Autodesk Fusion 360 part; units mm, degrees
note: some values were not read from the file. Set by a fixed rule: which sketch regions a step uses.
(part 9 of 59)
  spline S46 degree 5 poles (-3.7249, 43.2754) (-3.7256, 43.2728) (-3.7268, 43.2675) (-3.7287, 43.2596) (-3.7312, 43.2491) (-3.7343, 43.236) (-3.7374, 43.223) (-3.7405, 43.2099) (-3.7435, 43.1969) (-3.7466, 43.1839) (-3.7496, 43.171) (-3.7525, 43.158) (-3.7555, 43.1451) (-3.7584, 43.1323) (-3.7613, 43.1194) (-3.7642, 43.1066) (-3.767, 43.0938) (-3.7699, 43.081) (-3.7727, 43.0683) (-3.7755, 43.0556) (-3.7782, 43.0429) (-3.781, 43.0302) (-3.7837, 43.0176) (-3.7864, 43.005) (-3.7891, 42.9924) (-3.7917, 42.9799) (-3.7943, 42.9674) (-3.797, 42.9549) (-3.7995, 42.9424) (-3.8021, 42.93) (-3.8046, 42.9176) (-3.8071, 42.9053) (-3.8096, 42.8929) (-3.8121, 42.8806) (-3.8145, 42.8683) (-3.817, 42.8561) (-3.8194, 42.8439) (-3.8217, 42.8317) (-3.8241, 42.8195) (-3.8264, 42.8074) (-3.8288, 42.7953) (-3.831, 42.7832) (-3.8333, 42.7712) (-3.8356, 42.7592) (-3.8378, 42.7472) (-3.84, 42.7353) (-3.8422, 42.7233) (-3.8443, 42.7115) (-3.8464, 42.6996) (-3.8486, 42.6878) (-3.8507, 42.676) (-3.8527, 42.6643) (-3.8548, 42.6525) (-3.8568, 42.6409) (-3.8588, 42.6292) (-3.8608, 42.6176) (-3.8628, 42.606) (-3.8647, 42.5944) (-3.8666, 42.5829) (-3.8685, 42.5714) (-3.8704, 42.56) (-3.8722, 42.5486) (-3.8741, 42.5372) (-3.8759, 42.5258) (-3.8777, 42.5145) (-3.8795, 42.5032) (-3.8812, 42.492) (-3.8829, 42.4807) (-3.8846, 42.4696) (-3.8863, 42.4584) (-3.888, 42.4473) (-3.8896, 42.4362) (-3.8913, 42.4252) (-3.8929, 42.4142) (-3.8945, 42.4032) (-3.896, 42.3923) (-3.8976, 42.3814) (-3.8991, 42.3705) (-3.9006, 42.3597) (-3.9021, 42.3489) (-3.9035, 42.3382) (-3.905, 42.3274) (-3.9064, 42.3168) (-3.9078, 42.3061) (-3.9092, 42.2955) (-3.9106, 42.285) (-3.9119, 42.2744) (-3.9132, 42.264) (-3.9145, 42.2535) (-3.9158, 42.2431) (-3.9171, 42.2327) (-3.9183, 42.2224) (-3.9196, 42.2121) (-3.9208, 42.2018) (-3.922, 42.1916) (-3.9231, 42.1814) (-3.9243, 42.1713) (-3.9254, 42.1612) (-3.9265, 42.1512) (-3.9276, 42.1411) (-3.9287, 42.1312) (-3.9297, 42.1212) (-3.9308, 42.1113) (-3.9318, 42.1015) (-3.9328, 42.0917) (-3.9338, 42.0819) (-3.9348, 42.0722) (-3.9357, 42.0625) (-3.9366, 42.0529) (-3.9375, 42.0433) (-3.9384, 42.0337) (-3.9393, 42.0242) (-3.9402, 42.0147) (-3.941, 42.0053) (-3.9418, 41.9959) (-3.9426, 41.9866) (-3.9434, 41.9773) (-3.9442, 41.968) (-3.9449, 41.9588) (-3.9457, 41.9497) (-3.9464, 41.9406) (-3.9471, 41.9315) (-3.9478, 41.9225) (-3.9484, 41.9135) (-3.9491, 41.9045) (-3.9497, 41.8957) (-3.9503, 41.8868) (-3.9509, 41.878) (-3.9515, 41.8693) (-3.9521, 41.8606) (-3.9526, 41.8519) (-3.9532, 41.8433) (-3.9537, 41.8348) (-3.9542, 41.8263) (-3.9547, 41.8178) (-3.9552, 41.8094) (-3.9556, 41.801) (-3.9561, 41.7927) (-3.9565, 41.7845) (-3.9569, 41.7763) (-3.9573, 41.7681) (-3.9577, 41.76) (-3.9581, 41.7519) (-3.9584, 41.7439) (-3.9588, 41.736) (-3.9591, 41.7281) (-3.9594, 41.7202) (-3.9597, 41.7124) (-3.96, 41.7047) (-3.9603, 41.697) (-3.9605, 41.6893) (-3.9607, 41.6817) (-3.961, 41.6742) (-3.9612, 41.6667) (-3.9614, 41.6593) (-3.9616, 41.6519) (-3.9618, 41.6446) (-3.9619, 41.6374) (-3.9621, 41.6302) (-3.9622, 41.623) (-3.9623, 41.6159) (-3.9625, 41.6089) (-3.9626, 41.6019) (-3.9626, 41.595) (-3.9627, 41.5882) (-3.9628, 41.5814) (-3.9628, 41.5746) (-3.9629, 41.568) (-3.9629, 41.5613) (-3.9629, 41.5548) (-3.963, 41.5483) (-3.963, 41.5418) (-3.9629, 41.5355) (-3.9629, 41.5291) (-3.9629, 41.5229) (-3.9629, 41.5167) (-3.9628, 41.5106) (-3.9627, 41.5045) (-3.9627, 41.4985) (-3.9626, 41.4926) (-3.9625, 41.4867) (-3.9624, 41.4809) (-3.9623, 41.4752) (-3.9622, 41.4695) (-3.9621, 41.4639) (-3.962, 41.4584) (-3.9618, 41.4529) (-3.9617, 41.4475) (-3.9615, 41.4422) (-3.9614, 41.4369) (-3.9612, 41.4317) (-3.961, 41.4266) (-3.9609, 41.4215) (-3.9607, 41.4166) (-3.9605, 41.4117) (-3.9603, 41.4068) (-3.9601, 41.4021) (-3.9599, 41.3974) (-3.9597, 41.3928) (-3.9595, 41.3882) (-3.9593, 41.3838) (-3.959, 41.3794) (-3.9588, 41.3751) (-3.9586, 41.3709) (-3.9584, 41.3667) (-3.9581, 41.3626) (-3.9579, 41.3586) (-3.9577, 41.3547) (-3.9574, 41.3509) (-3.9572, 41.3472) (-3.9569, 41.3435) (-3.9567, 41.3399) (-3.9564, 41.3364) (-3.9562, 41.333) (-3.9559, 41.3297) (-3.9557, 41.3264) (-3.9555, 41.3233) (-3.9552, 41.3202) (-3.955, 41.3172) (-3.9547, 41.3144) (-3.9545, 41.3116) (-3.9543, 41.3089) (-3.954, 41.3063) (-3.9538, 41.3037) (-3.9536, 41.3013) (-3.9534, 41.299) (-3.9531, 41.2968) (-3.9529, 41.2946) (-3.9527, 41.2926) (-3.9525, 41.2907) (-3.9523, 41.2889) (-3.9522, 41.2871) (-3.952, 41.2855) (-3.9518, 41.284) (-3.9517, 41.2826) (-3.9515, 41.2813) (-3.9514, 41.2801) (-3.9512, 41.279) (-3.9511, 41.278) (-3.951, 41.2772) (-3.9509, 41.2764) (-3.9509, 41.2759) (-3.9508, 41.2756) (-3.9508, 41.2754) (-3.9508, 41.2753) knots -1 -1 -1 -1 -1 -1 -0.99583333 -0.99166667 -0.9875 -0.98333333 -0.97916667 -0.975 -0.97083333 -0.96666667 -0.9625 -0.95833333 -0.95416667 -0.95 -0.94583333 -0.94166667 -0.9375 -0.93333333 -0.92916667 -0.925 -0.92083333 -0.91666667 -0.9125 -0.90833333 -0.90416667 -0.9 -0.89583333 -0.89166667 -0.8875 -0.88333333 -0.87916667 -0.875 -0.87083333 -0.86666667 -0.8625 -0.85833333 -0.85416667 -0.85 -0.84583333 -0.84166667 -0.8375 -0.83333333 -0.82916667 -0.825 -0.82083333 -0.81666667 -0.8125 -0.80833333 -0.80416667 -0.8 -0.79583333 -0.79166667 -0.7875 -0.78333333 -0.77916667 -0.775 -0.77083333 -0.76666667 -0.7625 -0.75833333 -0.75416667 -0.75 -0.74583333 -0.74166667 -0.7375 -0.73333333 -0.72916667 -0.725 -0.72083333 -0.71666667 -0.7125 -0.70833333 -0.70416667 -0.7 -0.69583333 -0.69166667 -0.6875 -0.68333333 -0.67916667 -0.675 -0.67083333 -0.66666667 -0.6625 -0.65833333 -0.65416667 -0.65 -0.64583333 -0.64166667 -0.6375 -0.63333333 -0.62916667 -0.625 -0.62083333 -0.61666667 -0.6125 -0.60833333 -0.60416667 -0.6 -0.59583333 -0.59166667 -0.5875 -0.58333333 -0.57916667 -0.575 -0.57083333 -0.56666667 -0.5625 -0.55833333 -0.55416667 -0.55 -0.54583333 -0.54166667 -0.5375 -0.53333333 -0.52916667 -0.525 -0.52083333 -0.51666667 -0.5125 -0.50833333 -0.50416667 -0.5 -0.49583333 -0.49166667 -0.4875 -0.48333333 -0.47916667 -0.475 -0.47083333 -0.46666667 -0.4625 -0.45833333 -0.45416667 -0.45 -0.44583333 -0.44166667 -0.4375 -0.43333333 -0.42916667 -0.425 -0.42083333 -0.41666667 -0.4125 -0.40833333 -0.40416667 -0.4 -0.39583333 -0.39166667 -0.3875 -0.38333333 -0.37916667 -0.375 -0.37083333 -0.36666667 -0.3625 -0.35833333 -0.35416667 -0.35 -0.34583333 -0.34166667 -0.3375 -0.33333333 -0.32916667 -0.325 -0.32083333 -0.31666667 -0.3125 -0.30833333 -0.30416667 -0.3 -0.29583333 -0.29166667 -0.2875 -0.28333333 -0.27916667 -0.275 -0.27083333 -0.26666667 -0.2625 -0.25833333 -0.25416667 -0.25 -0.24583333 -0.24166667 -0.2375 -0.23333333 -0.22916667 -0.225 -0.22083333 -0.21666667 -0.2125 -0.20833333 -0.20416667 -0.2 -0.19583333 -0.19166667 -0.1875 -0.18333333 -0.17916667 -0.175 -0.17083333 -0.16666667 -0.1625 -0.15833333 -0.15416667 -0.15 -0.14583333 -0.14166667 -0.1375 -0.13333333 -0.12916667 -0.125 -0.12083333 -0.11666667 -0.1125 -0.10833333 -0.10416667 -0.1 -0.09583333 -0.09166667 -0.0875 -0.08333333 -0.07916667 -0.075 -0.07083333 -0.06666667 -0.0625 -0.05833333 -0.05416667 -0.05 -0.04583333 -0.04166667 -0.0375 -0.03333333 -0.02916667 -0.025 -0.02083333 -0.01666667 -0.0125 -0.00833333 -0.00416667 0 0 0 0 0 0
  spline S47 degree 5 poles (-21.1029, 35.2084) (-21.1018, 35.2059) (-21.0998, 35.2009) (-21.0967, 35.1934) (-21.0925, 35.1834) (-21.0873, 35.171) (-21.0822, 35.1586) (-21.077, 35.1462) (-21.0718, 35.1339) (-21.0666, 35.1217) (-21.0614, 35.1094) (-21.0562, 35.0972) (-21.051, 35.085) (-21.0458, 35.0729) (-21.0406, 35.0608) (-21.0354, 35.0487) (-21.0302, 35.0367) (-21.025, 35.0247) (-21.0198, 35.0127) (-21.0145, 35.0008) (-21.0093, 34.9889) (-21.0041, 34.9771) (-20.9989, 34.9653) (-20.9937, 34.9535) (-20.9884, 34.9417) (-20.9832, 34.93) (-20.978, 34.9184) (-20.9727, 34.9067) (-20.9675, 34.8951) (-20.9623, 34.8836) (-20.957, 34.8721) (-20.9518, 34.8606) (-20.9466, 34.8491) (-20.9413, 34.8377) (-20.9361, 34.8264) (-20.9308, 34.815) (-20.9256, 34.8037) (-20.9204, 34.7925) (-20.9151, 34.7812) (-20.9099, 34.7701) (-20.9046, 34.7589) (-20.8994, 34.7478) (-20.8942, 34.7367) (-20.8889, 34.7257) (-20.8837, 34.7147) (-20.8784, 34.7038) (-20.8732, 34.6928) (-20.868, 34.682) (-20.8627, 34.6711) (-20.8575, 34.6603) (-20.8523, 34.6496) (-20.847, 34.6388) (-20.8418, 34.6281) (-20.8366, 34.6175) (-20.8313, 34.6069) (-20.8261, 34.5963) (-20.8209, 34.5858) (-20.8157, 34.5753) (-20.8105, 34.5649) (-20.8052, 34.5544) (-20.8, 34.5441) (-20.7948, 34.5337) (-20.7896, 34.5235) (-20.7844, 34.5132) (-20.7792, 34.503) (-20.774, 34.4928) (-20.7688, 34.4827) (-20.7636, 34.4726) (-20.7584, 34.4625) (-20.7532, 34.4525) (-20.748, 34.4426) (-20.7429, 34.4326) (-20.7377, 34.4228) (-20.7325, 34.4129) (-20.7274, 34.4031) (-20.7222, 34.3933) (-20.717, 34.3836) (-20.7119, 34.3739) (-20.7067, 34.3643) (-20.7016, 34.3547) (-20.6965, 34.3451) (-20.6913, 34.3356) (-20.6862, 34.3261) (-20.6811, 34.3167) (-20.676, 34.3073) (-20.6709, 34.298) (-20.6658, 34.2887) (-20.6607, 34.2794) (-20.6556, 34.2702) (-20.6505, 34.261) (-20.6454, 34.2519) (-20.6404, 34.2428) (-20.6353, 34.2337) (-20.6303, 34.2247) (-20.6252, 34.2158) (-20.6202, 34.2068) (-20.6152, 34.198) (-20.6101, 34.1891) (-20.6051, 34.1803) (-20.6001, 34.1716) (-20.5951, 34.1629) (-20.5902, 34.1542) (-20.5852, 34.1456) (-20.5802, 34.1371) (-20.5753, 34.1285) (-20.5703, 34.1201) (-20.5654, 34.1116) (-20.5605, 34.1032) (-20.5555, 34.0949) (-20.5506, 34.0866) (-20.5457, 34.0783) (-20.5409, 34.0701) (-20.536, 34.0619) (-20.5311, 34.0538) (-20.5263, 34.0458) (-20.5214, 34.0377) (-20.5166, 34.0297) (-20.5118, 34.0218) (-20.507, 34.0139) (-20.5022, 34.0061) (-20.4974, 33.9983) (-20.4927, 33.9905) (-20.4879, 33.9828) (-20.4832, 33.9752) (-20.4784, 33.9676) (-20.4737, 33.96) (-20.469, 33.9525) (-20.4644, 33.945) (-20.4597, 33.9376) (-20.455, 33.9302) (-20.4504, 33.9229) (-20.4458, 33.9156) (-20.4412, 33.9084) (-20.4366, 33.9012) (-20.432, 33.8941) (-20.4274, 33.887) (-20.4229, 33.88) (-20.4184, 33.873) (-20.4139, 33.8661) (-20.4094, 33.8592) (-20.4049, 33.8523) (-20.4004, 33.8455) (-20.396, 33.8388) (-20.3916, 33.8321) (-20.3872, 33.8255) (-20.3828, 33.8189) (-20.3784, 33.8124) (-20.3741, 33.8059) (-20.3698, 33.7995) (-20.3655, 33.7931) (-20.3612, 33.7867) (-20.3569, 33.7805) (-20.3527, 33.7742) (-20.3484, 33.7681) (-20.3442, 33.7619) (-20.3401, 33.7559) (-20.3359, 33.7498) (-20.3318, 33.7439) (-20.3277, 33.738) (-20.3236, 33.7321) (-20.3195, 33.7263) (-20.3155, 33.7205) (-20.3115, 33.7148) (-20.3075, 33.7092) (-20.3035, 33.7036) (-20.2996, 33.6981) (-20.2956, 33.6926) (-20.2918, 33.6871) (-20.2879, 33.6818) (-20.2841, 33.6764) (-20.2802, 33.6712) (-20.2765, 33.666) (-20.2727, 33.6608) (-20.269, 33.6557) (-20.2653, 33.6507) (-20.2616, 33.6457) (-20.258, 33.6408) (-20.2544, 33.6359) (-20.2508, 33.6311) (-20.2472, 33.6263) (-20.2437, 33.6216) (-20.2402, 33.617) (-20.2368, 33.6124) (-20.2333, 33.6079) (-20.23, 33.6034) (-20.2266, 33.599) (-20.2233, 33.5947) (-20.22, 33.5904) (-20.2167, 33.5862) (-20.2135, 33.582) (-20.2103, 33.5779) (-20.2072, 33.5739) (-20.2041, 33.5699) (-20.201, 33.566) (-20.198, 33.5621) (-20.195, 33.5583) (-20.192, 33.5546) (-20.1891, 33.5509) (-20.1862, 33.5473) (-20.1834, 33.5437) (-20.1806, 33.5403) (-20.1778, 33.5368) (-20.1751, 33.5335) (-20.1724, 33.5302) (-20.1698, 33.527) (-20.1672, 33.5238) (-20.1647, 33.5207) (-20.1622, 33.5177) (-20.1597, 33.5148) (-20.1573, 33.5119) (-20.155, 33.509) (-20.1527, 33.5063) (-20.1504, 33.5036) (-20.1482, 33.501) (-20.1461, 33.4984) (-20.144, 33.496) (-20.1419, 33.4936) (-20.1399, 33.4912) (-20.138, 33.489) (-20.1361, 33.4868) (-20.1343, 33.4847) (-20.1325, 33.4826) (-20.1308, 33.4806) (-20.1291, 33.4787) (-20.1275, 33.4769) (-20.126, 33.4752) (-20.1245, 33.4735) (-20.123, 33.4719) (-20.1217, 33.4704) (-20.1204, 33.4689) (-20.1192, 33.4675) (-20.118, 33.4663) (-20.1169, 33.4651) (-20.1159, 33.4639) (-20.1149, 33.4629) (-20.114, 33.4619) (-20.1132, 33.461) (-20.1125, 33.4602) (-20.1118, 33.4595) (-20.1112, 33.4589) (-20.1107, 33.4583) (-20.1104, 33.458) (-20.1102, 33.4577) (-20.11, 33.4576) (-20.11, 33.4575) knots -1 -1 -1 -1 -1 -1 -0.99583333 -0.99166667 -0.9875 -0.98333333 -0.97916667 -0.975 -0.97083333 -0.96666667 -0.9625 -0.95833333 -0.95416667 -0.95 -0.94583333 -0.94166667 -0.9375 -0.93333333 -0.92916667 -0.925 -0.92083333 -0.91666667 -0.9125 -0.90833333 -0.90416667 -0.9 -0.89583333 -0.89166667 -0.8875 -0.88333333 -0.87916667 -0.875 -0.87083333 -0.86666667 -0.8625 -0.85833333 -0.85416667 -0.85 -0.84583333 -0.84166667 -0.8375 -0.83333333 -0.82916667 -0.825 -0.82083333 -0.81666667 -0.8125 -0.80833333 -0.80416667 -0.8 -0.79583333 -0.79166667 -0.7875 -0.78333333 -0.77916667 -0.775 -0.77083333 -0.76666667 -0.7625 -0.75833333 -0.75416667 -0.75 -0.74583333 -0.74166667 -0.7375 -0.73333333 -0.72916667 -0.725 -0.72083333 -0.71666667 -0.7125 -0.70833333 -0.70416667 -0.7 -0.69583333 -0.69166667 -0.6875 -0.68333333 -0.67916667 -0.675 -0.67083333 -0.66666667 -0.6625 -0.65833333 -0.65416667 -0.65 -0.64583333 -0.64166667 -0.6375 -0.63333333 -0.62916667 -0.625 -0.62083333 -0.61666667 -0.6125 -0.60833333 -0.60416667 -0.6 -0.59583333 -0.59166667 -0.5875 -0.58333333 -0.57916667 -0.575 -0.57083333 -0.56666667 -0.5625 -0.55833333 -0.55416667 -0.55 -0.54583333 -0.54166667 -0.5375 -0.53333333 -0.52916667 -0.525 -0.52083333 -0.51666667 -0.5125 -0.50833333 -0.50416667 -0.5 -0.49583333 -0.49166667 -0.4875 -0.48333333 -0.47916667 -0.475 -0.47083333 -0.46666667 -0.4625 -0.45833333 -0.45416667 -0.45 -0.44583333 -0.44166667 -0.4375 -0.43333333 -0.42916667 -0.425 -0.42083333 -0.41666667 -0.4125 -0.40833333 -0.40416667 -0.4 -0.39583333 -0.39166667 -0.3875 -0.38333333 -0.37916667 -0.375 -0.37083333 -0.36666667 -0.3625 -0.35833333 -0.35416667 -0.35 -0.34583333 -0.34166667 -0.3375 -0.33333333 -0.32916667 -0.325 -0.32083333 -0.31666667 -0.3125 -0.30833333 -0.30416667 -0.3 -0.29583333 -0.29166667 -0.2875 -0.28333333 -0.27916667 -0.275 -0.27083333 -0.26666667 -0.2625 -0.25833333 -0.25416667 -0.25 -0.24583333 -0.24166667 -0.2375 -0.23333333 -0.22916667 -0.225 -0.22083333 -0.21666667 -0.2125 -0.20833333 -0.20416667 -0.2 -0.19583333 -0.19166667 -0.1875 -0.18333333 -0.17916667 -0.175 -0.17083333 -0.16666667 -0.1625 -0.15833333 -0.15416667 -0.15 -0.14583333 -0.14166667 -0.1375 -0.13333333 -0.12916667 -0.125 -0.12083333 -0.11666667 -0.1125 -0.10833333 -0.10416667 -0.1 -0.09583333 -0.09166667 -0.0875 -0.08333333 -0.07916667 -0.075 -0.07083333 -0.06666667 -0.0625 -0.05833333 -0.05416667 -0.05 -0.04583333 -0.04166667 -0.0375 -0.03333333 -0.02916667 -0.025 -0.02083333 -0.01666667 -0.0125 -0.00833333 -0.00416667 0 0 0 0 0 0
  spline S48 degree 5 poles (-20.11, -8.4575) (-20.11, -8.4576) (-20.1102, -8.4577) (-20.1104, -8.458) (-20.1107, -8.4583) (-20.1112, -8.4589) (-20.1118, -8.4595) (-20.1125, -8.4602) (-20.1132, -8.461) (-20.114, -8.4619) (-20.1149, -8.4629) (-20.1159, -8.4639) (-20.1169, -8.4651) (-20.118, -8.4663) (-20.1192, -8.4675) (-20.1204, -8.4689) (-20.1217, -8.4704) (-20.123, -8.4719) (-20.1245, -8.4735) (-20.126, -8.4752) (-20.1275, -8.4769) (-20.1291, -8.4787) (-20.1308, -8.4806) (-20.1325, -8.4826) (-20.1343, -8.4847) (-20.1361, -8.4868) (-20.138, -8.489) (-20.1399, -8.4912) (-20.1419, -8.4936) (-20.144, -8.496) (-20.1461, -8.4984) (-20.1482, -8.501) (-20.1504, -8.5036) (-20.1527, -8.5063) (-20.155, -8.509) (-20.1573, -8.5119) (-20.1597, -8.5148) (-20.1622, -8.5177) (-20.1647, -8.5207) (-20.1672, -8.5238) (-20.1698, -8.527) (-20.1724, -8.5302) (-20.1751, -8.5335) (-20.1778, -8.5368) (-20.1806, -8.5403) (-20.1834, -8.5437) (-20.1862, -8.5473) (-20.1891, -8.5509) (-20.192, -8.5546) (-20.195, -8.5583) (-20.198, -8.5621) (-20.201, -8.566) (-20.2041, -8.5699) (-20.2072, -8.5739) (-20.2103, -8.5779) (-20.2135, -8.582) (-20.2167, -8.5862) (-20.22, -8.5904) (-20.2233, -8.5947) (-20.2266, -8.599) (-20.23, -8.6034) (-20.2333, -8.6079) (-20.2368, -8.6124) (-20.2402, -8.617) (-20.2437, -8.6216) (-20.2472, -8.6263) (-20.2508, -8.6311) (-20.2544, -8.6359) (-20.258, -8.6408) (-20.2616, -8.6457) (-20.2653, -8.6507) (-20.269, -8.6557) (-20.2727, -8.6608) (-20.2765, -8.666) (-20.2802, -8.6712) (-20.2841, -8.6764) (-20.2879, -8.6818) (-20.2918, -8.6871) (-20.2956, -8.6926) (-20.2996, -8.6981) (-20.3035, -8.7036) (-20.3075, -8.7092) (-20.3115, -8.7148) (-20.3155, -8.7205) (-20.3195, -8.7263) (-20.3236, -8.7321) (-20.3277, -8.738) (-20.3318, -8.7439) (-20.3359, -8.7498) (-20.3401, -8.7559) (-20.3442, -8.7619) (-20.3484, -8.7681) (-20.3527, -8.7742) (-20.3569, -8.7805) (-20.3612, -8.7867) (-20.3655, -8.7931) (-20.3698, -8.7995) (-20.3741, -8.8059) (-20.3784, -8.8124) (-20.3828, -8.8189) (-20.3872, -8.8255) (-20.3916, -8.8321) (-20.396, -8.8388) (-20.4004, -8.8455) (-20.4049, -8.8523) (-20.4094, -8.8592) (-20.4139, -8.8661) (-20.4184, -8.873) (-20.4229, -8.88) (-20.4274, -8.887) (-20.432, -8.8941) (-20.4366, -8.9012) (-20.4412, -8.9084) (-20.4458, -8.9156) (-20.4504, -8.9229) (-20.455, -8.9302) (-20.4597, -8.9376) (-20.4644, -8.945) (-20.469, -8.9525) (-20.4737, -8.96) (-20.4784, -8.9676) (-20.4832, -8.9752) (-20.4879, -8.9828) (-20.4927, -8.9905) (-20.4974, -8.9983) (-20.5022, -9.0061) (-20.507, -9.0139) (-20.5118, -9.0218) (-20.5166, -9.0297) (-20.5214, -9.0377) (-20.5263, -9.0458) (-20.5311, -9.0538) (-20.536, -9.0619) (-20.5409, -9.0701) (-20.5457, -9.0783) (-20.5506, -9.0866) (-20.5555, -9.0949) (-20.5605, -9.1032) (-20.5654, -9.1116) (-20.5703, -9.1201) (-20.5753, -9.1285) (-20.5802, -9.1371) (-20.5852, -9.1456) (-20.5902, -9.1542) (-20.5951, -9.1629) (-20.6001, -9.1716) (-20.6051, -9.1803) (-20.6101, -9.1891) (-20.6152, -9.198) (-20.6202, -9.2068) (-20.6252, -9.2158) (-20.6303, -9.2247) (-20.6353, -9.2337) (-20.6404, -9.2428) (-20.6454, -9.2519) (-20.6505, -9.261) (-20.6556, -9.2702) (-20.6607, -9.2794) (-20.6658, -9.2887) (-20.6709, -9.298) (-20.676, -9.3073) (-20.6811, -9.3167) (-20.6862, -9.3261) (-20.6913, -9.3356) (-20.6965, -9.3451) (-20.7016, -9.3547) (-20.7067, -9.3643) (-20.7119, -9.3739) (-20.717, -9.3836) (-20.7222, -9.3933) (-20.7274, -9.4031) (-20.7325, -9.4129) (-20.7377, -9.4228) (-20.7429, -9.4326) (-20.748, -9.4426) (-20.7532, -9.4525) (-20.7584, -9.4625) (-20.7636, -9.4726) (-20.7688, -9.4827) (-20.774, -9.4928) (-20.7792, -9.503) (-20.7844, -9.5132) (-20.7896, -9.5235) (-20.7948, -9.5337) (-20.8, -9.5441) (-20.8052, -9.5544) (-20.8105, -9.5649) (-20.8157, -9.5753) (-20.8209, -9.5858) (-20.8261, -9.5963) (-20.8313, -9.6069) (-20.8366, -9.6175) (-20.8418, -9.6281) (-20.847, -9.6388) (-20.8523, -9.6496) (-20.8575, -9.6603) (-20.8627, -9.6711) (-20.868, -9.682) (-20.8732, -9.6928) (-20.8784, -9.7038) (-20.8837, -9.7147) (-20.8889, -9.7257) (-20.8942, -9.7367) (-20.8994, -9.7478) (-20.9046, -9.7589) (-20.9099, -9.7701) (-20.9151, -9.7812) (-20.9204, -9.7925) (-20.9256, -9.8037) (-20.9308, -9.815) (-20.9361, -9.8264) (-20.9413, -9.8377) (-20.9466, -9.8491) (-20.9518, -9.8606) (-20.957, -9.8721) (-20.9623, -9.8836) (-20.9675, -9.8951) (-20.9727, -9.9067) (-20.978, -9.9184) (-20.9832, -9.93) (-20.9884, -9.9417) (-20.9937, -9.9535) (-20.9989, -9.9653) (-21.0041, -9.9771) (-21.0093, -9.9889) (-21.0145, -10.0008) (-21.0198, -10.0127) (-21.025, -10.0247) (-21.0302, -10.0367) (-21.0354, -10.0487) (-21.0406, -10.0608) (-21.0458, -10.0729) (-21.051, -10.085) (-21.0562, -10.0972) (-21.0614, -10.1094) (-21.0666, -10.1217) (-21.0718, -10.1339) (-21.077, -10.1462) (-21.0822, -10.1586) (-21.0873, -10.171) (-21.0925, -10.1834) (-21.0967, -10.1934) (-21.0998, -10.2009) (-21.1018, -10.2059) (-21.1029, -10.2084) knots 0 0 0 0 0 0 0.00416667 0.00833333 0.0125 0.01666667 0.02083333 0.025 0.02916667 0.03333333 0.0375 0.04166667 0.04583333 0.05 0.05416667 0.05833333 0.0625 0.06666667 0.07083333 0.075 0.07916667 0.08333333 0.0875 0.09166667 0.09583333 0.1 0.10416667 0.10833333 0.1125 0.11666667 0.12083333 0.125 0.12916667 0.13333333 0.1375 0.14166667 0.14583333 0.15 0.15416667 0.15833333 0.1625 0.16666667 0.17083333 0.175 0.17916667 0.18333333 0.1875 0.19166667 0.19583333 0.2 0.20416667 0.20833333 0.2125 0.21666667 0.22083333 0.225 0.22916667 0.23333333 0.2375 0.24166667 0.24583333 0.25 0.25416667 0.25833333 0.2625 0.26666667 0.27083333 0.275 0.27916667 0.28333333 0.2875 0.29166667 0.29583333 0.3 0.30416667 0.30833333 0.3125 0.31666667 0.32083333 0.325 0.32916667 0.33333333 0.3375 0.34166667 0.34583333 0.35 0.35416667 0.35833333 0.3625 0.36666667 0.37083333 0.375 0.37916667 0.38333333 0.3875 0.39166667 0.39583333 0.4 0.40416667 0.40833333 0.4125 0.41666667 0.42083333 0.425 0.42916667 0.43333333 0.4375 0.44166667 0.44583333 0.45 0.45416667 0.45833333 0.4625 0.46666667 0.47083333 0.475 0.47916667 0.48333333 0.4875 0.49166667 0.49583333 0.5 0.50416667 0.50833333 0.5125 0.51666667 0.52083333 0.525 0.52916667 0.53333333 0.5375 0.54166667 0.54583333 0.55 0.55416667 0.55833333 0.5625 0.56666667 0.57083333 0.575 0.57916667 0.58333333 0.5875 0.59166667 0.59583333 0.6 0.60416667 0.60833333 0.6125 0.61666667 0.62083333 0.625 0.62916667 0.63333333 0.6375 0.64166667 0.64583333 0.65 0.65416667 0.65833333 0.6625 0.66666667 0.67083333 0.675 0.67916667 0.68333333 0.6875 0.69166667 0.69583333 0.7 0.70416667 0.70833333 0.7125 0.71666667 0.72083333 0.725 0.72916667 0.73333333 0.7375 0.74166667 0.74583333 0.75 0.75416667 0.75833333 0.7625 0.76666667 0.77083333 0.775 0.77916667 0.78333333 0.7875 0.79166667 0.79583333 0.8 0.80416667 0.80833333 0.8125 0.81666667 0.82083333 0.825 0.82916667 0.83333333 0.8375 0.84166667 0.84583333 0.85 0.85416667 0.85833333 0.8625 0.86666667 0.87083333 0.875 0.87916667 0.88333333 0.8875 0.89166667 0.89583333 0.9 0.90416667 0.90833333 0.9125 0.91666667 0.92083333 0.925 0.92916667 0.93333333 0.9375 0.94166667 0.94583333 0.95 0.95416667 0.95833333 0.9625 0.96666667 0.97083333 0.975 0.97916667 0.98333333 0.9875 0.99166667 0.99583333 1 1 1 1 1 1
  line L118 (-8.0125, 40.1109) -> (-8.0945, 40.3937)
  arc A63 (-5.9675, 42.9202) -> (-6.9214, 42.7174) centre (0, 12.5) ccw
  line L119 (-6.9368, 40.7039) -> (-6.8665, 40.418)
  arc A64 (-9.7471, 39.5473) -> (-10.8547, 39.1221) centre (0, 12.5) ccw
  spline S49 degree 5 poles (-10.9662, 39.3955) (-10.9662, 39.3956) (-10.9663, 39.3958) (-10.9664, 39.3961) (-10.9666, 39.3966) (-10.9669, 39.3973) (-10.9672, 39.3981) (-10.9676, 39.399) (-10.9681, 39.4) (-10.9685, 39.4011) (-10.9691, 39.4023) (-10.9696, 39.4036) (-10.9702, 39.405) (-10.9709, 39.4065) (-10.9716, 39.408) (-10.9724, 39.4097) (-10.9731, 39.4115) (-10.974, 39.4134) (-10.9749, 39.4153) (-10.9758, 39.4173) (-10.9768, 39.4195) (-10.9778, 39.4217) (-10.9788, 39.424) (-10.9799, 39.4263) (-10.9811, 39.4288) (-10.9823, 39.4313) (-10.9835, 39.4339) (-10.9848, 39.4366) (-10.9861, 39.4394) (-10.9875, 39.4423) (-10.9889, 39.4452) (-10.9903, 39.4482) (-10.9918, 39.4513) (-10.9934, 39.4544) (-10.9949, 39.4577) (-10.9966, 39.461) (-10.9982, 39.4643) (-10.9999, 39.4678) (-11.0017, 39.4713) (-11.0035, 39.4748) (-11.0053, 39.4785) (-11.0072, 39.4822) (-11.0091, 39.486) (-11.0111, 39.4898) (-11.0131, 39.4937) (-11.0151, 39.4977) (-11.0172, 39.5017) (-11.0193, 39.5058) (-11.0215, 39.51) (-11.0237, 39.5142) (-11.0259, 39.5185) (-11.0282, 39.5228) (-11.0306, 39.5272) (-11.0329, 39.5317) (-11.0353, 39.5362) (-11.0378, 39.5408) (-11.0403, 39.5454) (-11.0428, 39.5501) (-11.0454, 39.5549) (-11.048, 39.5597) (-11.0507, 39.5645) (-11.0534, 39.5694) (-11.0561, 39.5744) (-11.0589, 39.5794) (-11.0617, 39.5845) (-11.0646, 39.5896) (-11.0675, 39.5948) (-11.0704, 39.6) (-11.0734, 39.6053) (-11.0764, 39.6106) (-11.0795, 39.616) (-11.0826, 39.6214) (-11.0857, 39.6269) (-11.0889, 39.6324) (-11.0921, 39.638) (-11.0954, 39.6436) (-11.0987, 39.6493) (-11.102, 39.655) (-11.1054, 39.6608) (-11.1088, 39.6666) (-11.1123, 39.6725) (-11.1158, 39.6784) (-11.1193, 39.6843) (-11.1229, 39.6903) (-11.1265, 39.6963) (-11.1301, 39.7024) (-11.1338, 39.7085) (-11.1376, 39.7147) (-11.1413, 39.7209) (-11.1451, 39.7271) (-11.149, 39.7334) (-11.1529, 39.7397) (-11.1568, 39.7461) (-11.1608, 39.7525) (-11.1648, 39.759) (-11.1688, 39.7654) (-11.1729, 39.772) (-11.177, 39.7785) (-11.1812, 39.7851) (-11.1854, 39.7918) (-11.1896, 39.7985) (-11.1939, 39.8052) (-11.1982, 39.8119) (-11.2025, 39.8187) (-11.2069, 39.8256) (-11.2113, 39.8324) (-11.2158, 39.8393) (-11.2203, 39.8463) (-11.2248, 39.8533) (-11.2294, 39.8603) (-11.234, 39.8673) (-11.2387, 39.8744) (-11.2434, 39.8815) (-11.2481, 39.8887) (-11.2529, 39.8958) (-11.2577, 39.9031) (-11.2625, 39.9103) (-11.2674, 39.9176) (-11.2723, 39.9249) (-11.2773, 39.9323) (-11.2823, 39.9396) (-11.2873, 39.947) (-11.2924, 39.9545) (-11.2975, 39.962) (-11.3026, 39.9695) (-11.3078, 39.977) (-11.313, 39.9846) (-11.3183, 39.9922) (-11.3235, 39.9998) (-11.3289, 40.0074) (-11.3342, 40.0151) (-11.3396, 40.0228) (-11.3451, 40.0306) (-11.3506, 40.0384) (-11.3561, 40.0462) (-11.3616, 40.054) (-11.3672, 40.0618) (-11.3728, 40.0697) (-11.3785, 40.0776) (-11.3842, 40.0856) (-11.3899, 40.0936) (-11.3957, 40.1015) (-11.4015, 40.1096) (-11.4074, 40.1176) (-11.4132, 40.1257) (-11.4192, 40.1338) (-11.4251, 40.1419) (-11.4311, 40.1501) (-11.4371, 40.1582) (-11.4432, 40.1665) (-11.4493, 40.1747) (-11.4554, 40.1829) (-11.4616, 40.1912) (-11.4678, 40.1995) (-11.4741, 40.2078) (-11.4803, 40.2162) (-11.4867, 40.2246) (-11.493, 40.233) (-11.4994, 40.2414) (-11.5058, 40.2498) (-11.5123, 40.2583) (-11.5188, 40.2668) (-11.5253, 40.2753) (-11.5319, 40.2838) (-11.5385, 40.2924) (-11.5452, 40.301) (-11.5518, 40.3096) (-11.5585, 40.3182) (-11.5653, 40.3268) (-11.5721, 40.3355) (-11.5789, 40.3442) (-11.5858, 40.3529) (-11.5927, 40.3616) (-11.5996, 40.3704) (-11.6065, 40.3791) (-11.6135, 40.3879) (-11.6206, 40.3967) (-11.6276, 40.4055) (-11.6348, 40.4144) (-11.6419, 40.4233) (-11.6491, 40.4322) (-11.6563, 40.4411) (-11.6635, 40.45) (-11.6708, 40.4589) (-11.6781, 40.4679) (-11.6855, 40.4769) (-11.6929, 40.4859) (-11.7003, 40.4949) (-11.7078, 40.5039) (-11.7153, 40.513) (-11.7228, 40.5221) (-11.7303, 40.5312) (-11.7379, 40.5403) (-11.7456, 40.5494) (-11.7532, 40.5585) (-11.7609, 40.5677) (-11.7687, 40.5769) (-11.7765, 40.5861) (-11.7843, 40.5953) (-11.7921, 40.6045) (-11.8, 40.6137) (-11.8079, 40.623) (-11.8158, 40.6323) (-11.8238, 40.6416) (-11.8318, 40.6509) (-11.8399, 40.6602) (-11.848, 40.6695) (-11.8561, 40.6789) (-11.8643, 40.6882) (-11.8724, 40.6976) (-11.8807, 40.707) (-11.8889, 40.7164) (-11.8972, 40.7259) (-11.9055, 40.7353) (-11.9139, 40.7447) (-11.9223, 40.7542) (-11.9307, 40.7637) (-11.9392, 40.7732) (-11.9477, 40.7827) (-11.9562, 40.7922) (-11.9648, 40.8018) (-11.9734, 40.8113) (-11.982, 40.8209) (-11.9907, 40.8305) (-11.9994, 40.84) (-12.0081, 40.8496) (-12.0169, 40.8593) (-12.0257, 40.8689) (-12.0345, 40.8785) (-12.0434, 40.8882) (-12.0523, 40.8978) (-12.0613, 40.9075) (-12.0702, 40.9172) (-12.0792, 40.9269) (-12.0883, 40.9366) (-12.0973, 40.9464) (-12.1065, 40.9561) (-12.1156, 40.9658) (-12.1248, 40.9756) (-12.134, 40.9854) (-12.1432, 40.9951) (-12.1506, 41.003) (-12.1562, 41.0089) (-12.16, 41.0128) (-12.1618, 41.0147) knots 0 0 0 0 0 0 0.00416667 0.00833333 0.0125 0.01666667 0.02083333 0.025 0.02916667 0.03333333 0.0375 0.04166667 0.04583333 0.05 0.05416667 0.05833333 0.0625 0.06666667 0.07083333 0.075 0.07916667 0.08333333 0.0875 0.09166667 0.09583333 0.1 0.10416667 0.10833333 0.1125 0.11666667 0.12083333 0.125 0.12916667 0.13333333 0.1375 0.14166667 0.14583333 0.15 0.15416667 0.15833333 0.1625 0.16666667 0.17083333 0.175 0.17916667 0.18333333 0.1875 0.19166667 0.19583333 0.2 0.20416667 0.20833333 0.2125 0.21666667 0.22083333 0.225 0.22916667 0.23333333 0.2375 0.24166667 0.24583333 0.25 0.25416667 0.25833333 0.2625 0.26666667 0.27083333 0.275 0.27916667 0.28333333 0.2875 0.29166667 0.29583333 0.3 0.30416667 0.30833333 0.3125 0.31666667 0.32083333 0.325 0.32916667 0.33333333 0.3375 0.34166667 0.34583333 0.35 0.35416667 0.35833333 0.3625 0.36666667 0.37083333 0.375 0.37916667 0.38333333 0.3875 0.39166667 0.39583333 0.4 0.40416667 0.40833333 0.4125 0.41666667 0.42083333 0.425 0.42916667 0.43333333 0.4375 0.44166667 0.44583333 0.45 0.45416667 0.45833333 0.4625 0.46666667 0.47083333 0.475 0.47916667 0.48333333 0.4875 0.49166667 0.49583333 0.5 0.50416667 0.50833333 0.5125 0.51666667 0.52083333 0.525 0.52916667 0.53333333 0.5375 0.54166667 0.54583333 0.55 0.55416667 0.55833333 0.5625 0.56666667 0.57083333 0.575 0.57916667 0.58333333 0.5875 0.59166667 0.59583333 0.6 0.60416667 0.60833333 0.6125 0.61666667 0.62083333 0.625 0.62916667 0.63333333 0.6375 0.64166667 0.64583333 0.65 0.65416667 0.65833333 0.6625 0.66666667 0.67083333 0.675 0.67916667 0.68333333 0.6875 0.69166667 0.69583333 0.7 0.70416667 0.70833333 0.7125 0.71666667 0.72083333 0.725 0.72916667 0.73333333 0.7375 0.74166667 0.74583333 0.75 0.75416667 0.75833333 0.7625 0.76666667 0.77083333 0.775 0.77916667 0.78333333 0.7875 0.79166667 0.79583333 0.8 0.80416667 0.80833333 0.8125 0.81666667 0.82083333 0.825 0.82916667 0.83333333 0.8375 0.84166667 0.84583333 0.85 0.85416667 0.85833333 0.8625 0.86666667 0.87083333 0.875 0.87916667 0.88333333 0.8875 0.89166667 0.89583333 0.9 0.90416667 0.90833333 0.9125 0.91666667 0.92083333 0.925 0.92916667 0.93333333 0.9375 0.94166667 0.94583333 0.95 0.95416667 0.95833333 0.9625 0.96666667 0.97083333 0.975 0.97916667 0.98333333 0.9875 0.99166667 0.99583333 1 1 1 1 1 1
  spline S50 degree 5 poles (-16.3184, 36.5278) (-16.3185, 36.5279) (-16.3186, 36.5281) (-16.3188, 36.5283) (-16.3191, 36.5287) (-16.3195, 36.5294) (-16.32, 36.5301) (-16.3206, 36.5309) (-16.3212, 36.5317) (-16.3219, 36.5327) (-16.3227, 36.5338) (-16.3235, 36.535) (-16.3244, 36.5362) (-16.3253, 36.5375) (-16.3263, 36.5389) (-16.3274, 36.5404) (-16.3286, 36.542) (-16.3298, 36.5436) (-16.331, 36.5453) (-16.3324, 36.5471) (-16.3338, 36.549) (-16.3352, 36.551) (-16.3367, 36.553) (-16.3383, 36.5551) (-16.3399, 36.5572) (-16.3416, 36.5595) (-16.3434, 36.5618) (-16.3452, 36.5641) (-16.3471, 36.5666) (-16.349, 36.5691) (-16.351, 36.5717) (-16.353, 36.5743) (-16.3551, 36.577) (-16.3573, 36.5798) (-16.3595, 36.5826) (-16.3618, 36.5855) (-16.3641, 36.5884) (-16.3665, 36.5914) (-16.3689, 36.5945) (-16.3714, 36.5976) (-16.374, 36.6008) (-16.3766, 36.604) (-16.3792, 36.6073) (-16.3819, 36.6107) (-16.3847, 36.6141) (-16.3875, 36.6176) (-16.3904, 36.6211) (-16.3933, 36.6246) (-16.3963, 36.6283) (-16.3994, 36.6319) (-16.4024, 36.6356) (-16.4056, 36.6394) (-16.4088, 36.6432) (-16.412, 36.6471) (-16.4153, 36.651) (-16.4187, 36.655) (-16.4221, 36.659) (-16.4256, 36.6631) (-16.4291, 36.6672) (-16.4326, 36.6713) (-16.4362, 36.6755) (-16.4399, 36.6798) (-16.4436, 36.6841) (-16.4474, 36.6884) (-16.4512, 36.6928) (-16.455, 36.6972) (-16.459, 36.7017) (-16.4629, 36.7062) (-16.4669, 36.7107) (-16.471, 36.7153) (-16.4751, 36.7199) (-16.4793, 36.7246) (-16.4835, 36.7293) (-16.4877, 36.734) (-16.492, 36.7388) (-16.4964, 36.7436) (-16.5008, 36.7485) (-16.5053, 36.7534) (-16.5098, 36.7583) (-16.5143, 36.7633) (-16.5189, 36.7683) (-16.5236, 36.7733) (-16.5282, 36.7784) (-16.533, 36.7835) (-16.5378, 36.7887) (-16.5426, 36.7939) (-16.5475, 36.7991) (-16.5524, 36.8043) (-16.5574, 36.8096) (-16.5624, 36.8149) (-16.5675, 36.8203) (-16.5726, 36.8257) (-16.5778, 36.8311) (-16.583, 36.8365) (-16.5882, 36.842) (-16.5935, 36.8475) (-16.5989, 36.853) (-16.6043, 36.8586) (-16.6097, 36.8642) (-16.6152, 36.8698) (-16.6207, 36.8755) (-16.6263, 36.8812) (-16.6319, 36.8869) (-16.6376, 36.8926) (-16.6433, 36.8984) (-16.6491, 36.9042) (-16.6549, 36.91) (-16.6607, 36.9159) (-16.6666, 36.9218) (-16.6725, 36.9277) (-16.6785, 36.9336) (-16.6845, 36.9395) (-16.6906, 36.9455) (-16.6967, 36.9515) (-16.7029, 36.9576) (-16.7091, 36.9636) (-16.7153, 36.9697) (-16.7216, 36.9758) (-16.7279, 36.982) (-16.7343, 36.9881) (-16.7407, 36.9943) (-16.7472, 37.0005) (-16.7537, 37.0067) (-16.7602, 37.013) (-16.7668, 37.0192) (-16.7735, 37.0255) (-16.7801, 37.0319) (-16.7869, 37.0382) (-16.7936, 37.0446) (-16.8004, 37.0509) (-16.8073, 37.0573) (-16.8142, 37.0638) (-16.8211, 37.0702) (-16.8281, 37.0767) (-16.8351, 37.0831) (-16.8421, 37.0897) (-16.8492, 37.0962) (-16.8564, 37.1027) (-16.8636, 37.1093) (-16.8708, 37.1159) (-16.8781, 37.1225) (-16.8854, 37.1291) (-16.8927, 37.1357) (-16.9001, 37.1424) (-16.9075, 37.1491) (-16.915, 37.1558) (-16.9225, 37.1625) (-16.9301, 37.1692) (-16.9377, 37.1759) (-16.9453, 37.1827) (-16.953, 37.1895) (-16.9607, 37.1963) (-16.9685, 37.2031) (-16.9763, 37.2099) (-16.9841, 37.2168) (-16.992, 37.2236) (-16.9999, 37.2305) (-17.0079, 37.2374) (-17.0159, 37.2443) (-17.0239, 37.2512) (-17.032, 37.2582) (-17.0401, 37.2651) (-17.0483, 37.2721) (-17.0565, 37.2791) (-17.0647, 37.2861) (-17.073, 37.2931) (-17.0813, 37.3001) (-17.0897, 37.3071) (-17.0981, 37.3142) (-17.1065, 37.3212) (-17.115, 37.3283) (-17.1235, 37.3354) (-17.1321, 37.3425) (-17.1407, 37.3496) (-17.1493, 37.3568) (-17.158, 37.3639) (-17.1667, 37.3711) (-17.1754, 37.3782) (-17.1842, 37.3854) (-17.1931, 37.3926) (-17.2019, 37.3998) (-17.2108, 37.407) (-17.2198, 37.4142) (-17.2288, 37.4215) (-17.2378, 37.4287) (-17.2469, 37.436) (-17.2559, 37.4432) (-17.2651, 37.4505) (-17.2743, 37.4578) (-17.2835, 37.4651) (-17.2927, 37.4724) (-17.302, 37.4797) (-17.3113, 37.4871) (-17.3207, 37.4944) (-17.3301, 37.5017) (-17.3395, 37.5091) (-17.349, 37.5165) (-17.3585, 37.5238) (-17.3681, 37.5312) (-17.3777, 37.5386) (-17.3873, 37.546) (-17.397, 37.5534) (-17.4067, 37.5609) (-17.4164, 37.5683) (-17.4262, 37.5757) (-17.436, 37.5832) (-17.4458, 37.5906) (-17.4557, 37.5981) (-17.4657, 37.6055) (-17.4756, 37.613) (-17.4856, 37.6205) (-17.4956, 37.628) (-17.5057, 37.6355) (-17.5158, 37.643) (-17.526, 37.6505) (-17.5361, 37.658) (-17.5464, 37.6655) (-17.5566, 37.6731) (-17.5669, 37.6806) (-17.5772, 37.6881) (-17.5876, 37.6957) (-17.598, 37.7032) (-17.6084, 37.7108) (-17.6189, 37.7184) (-17.6294, 37.7259) (-17.6399, 37.7335) (-17.6505, 37.7411) (-17.6611, 37.7487) (-17.6718, 37.7563) (-17.6825, 37.7639) (-17.6932, 37.7715) (-17.7039, 37.7791) (-17.7147, 37.7867) (-17.7256, 37.7943) (-17.7364, 37.8019) (-17.7473, 37.8096) (-17.7583, 37.8172) (-17.7692, 37.8248) (-17.7802, 37.8325) (-17.7913, 37.8401) (-17.8023, 37.8477) (-17.8112, 37.8539) (-17.8179, 37.8584) (-17.8224, 37.8615) (-17.8246, 37.863) knots 0 0 0 0 0 0 0.00416667 0.00833333 0.0125 0.01666667 0.02083333 0.025 0.02916667 0.03333333 0.0375 0.04166667 0.04583333 0.05 0.05416667 0.05833333 0.0625 0.06666667 0.07083333 0.075 0.07916667 0.08333333 0.0875 0.09166667 0.09583333 0.1 0.10416667 0.10833333 0.1125 0.11666667 0.12083333 0.125 0.12916667 0.13333333 0.1375 0.14166667 0.14583333 0.15 0.15416667 0.15833333 0.1625 0.16666667 0.17083333 0.175 0.17916667 0.18333333 0.1875 0.19166667 0.19583333 0.2 0.20416667 0.20833333 0.2125 0.21666667 0.22083333 0.225 0.22916667 0.23333333 0.2375 0.24166667 0.24583333 0.25 0.25416667 0.25833333 0.2625 0.26666667 0.27083333 0.275 0.27916667 0.28333333 0.2875 0.29166667 0.29583333 0.3 0.30416667 0.30833333 0.3125 0.31666667 0.32083333 0.325 0.32916667 0.33333333 0.3375 0.34166667 0.34583333 0.35 0.35416667 0.35833333 0.3625 0.36666667 0.37083333 0.375 0.37916667 0.38333333 0.3875 0.39166667 0.39583333 0.4 0.40416667 0.40833333 0.4125 0.41666667 0.42083333 0.425 0.42916667 0.43333333 0.4375 0.44166667 0.44583333 0.45 0.45416667 0.45833333 0.4625 0.46666667 0.47083333 0.475 0.47916667 0.48333333 0.4875 0.49166667 0.49583333 0.5 0.50416667 0.50833333 0.5125 0.51666667 0.52083333 0.525 0.52916667 0.53333333 0.5375 0.54166667 0.54583333 0.55 0.55416667 0.55833333 0.5625 0.56666667 0.57083333 0.575 0.57916667 0.58333333 0.5875 0.59166667 0.59583333 0.6 0.60416667 0.60833333 0.6125 0.61666667 0.62083333 0.625 0.62916667 0.63333333 0.6375 0.64166667 0.64583333 0.65 0.65416667 0.65833333 0.6625 0.66666667 0.67083333 0.675 0.67916667 0.68333333 0.6875 0.69166667 0.69583333 0.7 0.70416667 0.70833333 0.7125 0.71666667 0.72083333 0.725 0.72916667 0.73333333 0.7375 0.74166667 0.74583333 0.75 0.75416667 0.75833333 0.7625 0.76666667 0.77083333 0.775 0.77916667 0.78333333 0.7875 0.79166667 0.79583333 0.8 0.80416667 0.80833333 0.8125 0.81666667 0.82083333 0.825 0.82916667 0.83333333 0.8375 0.84166667 0.84583333 0.85 0.85416667 0.85833333 0.8625 0.86666667 0.87083333 0.875 0.87916667 0.88333333 0.8875 0.89166667 0.89583333 0.9 0.90416667 0.90833333 0.9125 0.91666667 0.92083333 0.925 0.92916667 0.93333333 0.9375 0.94166667 0.94583333 0.95 0.95416667 0.95833333 0.9625 0.96666667 0.97083333 0.975 0.97916667 0.98333333 0.9875 0.99166667 0.99583333 1 1 1 1 1 1
  spline S51 degree 5 poles (-18.6136, 37.2898) (-18.6128, 37.2872) (-18.6113, 37.282) (-18.609, 37.2743) (-18.6059, 37.2639) (-18.6021, 37.251) (-18.5982, 37.2382) (-18.5943, 37.2253) (-18.5905, 37.2125) (-18.5866, 37.1998) (-18.5827, 37.1871) (-18.5788, 37.1744) (-18.5749, 37.1617) (-18.571, 37.1491) (-18.5671, 37.1365) (-18.5632, 37.124) (-18.5593, 37.1115) (-18.5553, 37.099) (-18.5514, 37.0866) (-18.5475, 37.0742) (-18.5435, 37.0618) (-18.5395, 37.0495) (-18.5356, 37.0372) (-18.5316, 37.0249) (-18.5277, 37.0127) (-18.5237, 37.0005) (-18.5197, 36.9884) (-18.5157, 36.9762) (-18.5117, 36.9642) (-18.5077, 36.9521) (-18.5037, 36.9401) (-18.4997, 36.9281) (-18.4957, 36.9162) (-18.4917, 36.9043) (-18.4877, 36.8925) (-18.4836, 36.8806) (-18.4796, 36.8689) (-18.4756, 36.8571) (-18.4715, 36.8454) (-18.4675, 36.8337) (-18.4634, 36.8221) (-18.4594, 36.8105) (-18.4553, 36.799) (-18.4513, 36.7874) (-18.4472, 36.776) (-18.4431, 36.7645) (-18.4391, 36.7531) (-18.435, 36.7417) (-18.4309, 36.7304) (-18.4269, 36.7191) (-18.4228, 36.7079) (-18.4187, 36.6967) (-18.4146, 36.6855) (-18.4105, 36.6744) (-18.4064, 36.6633) (-18.4023, 36.6522) (-18.3982, 36.6412) (-18.3941, 36.6302) (-18.39, 36.6193) (-18.3859, 36.6084) (-18.3818, 36.5975) (-18.3777, 36.5867) (-18.3736, 36.5759) (-18.3695, 36.5652) (-18.3654, 36.5545) (-18.3613, 36.5438) (-18.3572, 36.5332) (-18.3531, 36.5226) (-18.349, 36.5121) (-18.3449, 36.5016) (-18.3408, 36.4911) (-18.3366, 36.4807) (-18.3325, 36.4703) (-18.3284, 36.46) (-18.3243, 36.4497) (-18.3202, 36.4395) (-18.3161, 36.4292) (-18.312, 36.4191) (-18.3079, 36.409) (-18.3038, 36.3989) (-18.2996, 36.3888) (-18.2955, 36.3788) (-18.2914, 36.3689) (-18.2873, 36.359) (-18.2832, 36.3491) (-18.2791, 36.3393) (-18.275, 36.3295) (-18.2709, 36.3197) (-18.2668, 36.31) (-18.2627, 36.3004) (-18.2587, 36.2907) (-18.2546, 36.2812) (-18.2505, 36.2716) (-18.2464, 36.2622) (-18.2423, 36.2527) (-18.2383, 36.2433) (-18.2342, 36.234) (-18.2301, 36.2247) (-18.226, 36.2154) (-18.222, 36.2062) (-18.2179, 36.197) (-18.2139, 36.1879) (-18.2098, 36.1788) (-18.2058, 36.1697) (-18.2018, 36.1607) (-18.1977, 36.1518) (-18.1937, 36.1429) (-18.1897, 36.134) (-18.1857, 36.1252) (-18.1816, 36.1165) (-18.1776, 36.1077) (-18.1736, 36.0991) (-18.1696, 36.0904) (-18.1657, 36.0818) (-18.1617, 36.0733) (-18.1577, 36.0648) (-18.1537, 36.0564) (-18.1498, 36.048) (-18.1458, 36.0396) (-18.1419, 36.0313) (-18.1379, 36.0231) (-18.134, 36.0149) (-18.1301, 36.0067) (-18.1262, 35.9986) (-18.1223, 35.9905) (-18.1184, 35.9825) (-18.1145, 35.9746) (-18.1106, 35.9666) (-18.1068, 35.9588) (-18.1029, 35.951) (-18.0991, 35.9432) (-18.0952, 35.9355) (-18.0914, 35.9278) (-18.0876, 35.9202) (-18.0838, 35.9126) (-18.08, 35.9051) (-18.0762, 35.8976) (-18.0724, 35.8902) (-18.0687, 35.8828) (-18.0649, 35.8755) (-18.0612, 35.8683) (-18.0575, 35.861) (-18.0538, 35.8539) (-18.0501, 35.8468) (-18.0464, 35.8397) (-18.0427, 35.8327) (-18.039, 35.8257) (-18.0354, 35.8188) (-18.0318, 35.812) (-18.0282, 35.8052) (-18.0246, 35.7984) (-18.021, 35.7918) (-18.0174, 35.7851) (-18.0139, 35.7785) (-18.0103, 35.772) (-18.0068, 35.7655) (-18.0033, 35.7591) (-17.9998, 35.7527) (-17.9963, 35.7464) (-17.9929, 35.7402) (-17.9895, 35.734) (-17.986, 35.7278) (-17.9826, 35.7217) (-17.9793, 35.7157) (-17.9759, 35.7097) (-17.9726, 35.7038) (-17.9692, 35.6979) (-17.9659, 35.6921) (-17.9627, 35.6864) (-17.9594, 35.6807) (-17.9562, 35.6751) (-17.9529, 35.6695) (-17.9497, 35.664) (-17.9466, 35.6585) (-17.9434, 35.6531) (-17.9403, 35.6478) (-17.9372, 35.6425) (-17.9341, 35.6373) (-17.931, 35.6321) (-17.928, 35.627) (-17.925, 35.622) (-17.922, 35.617) (-17.9191, 35.6121) (-17.9161, 35.6072) (-17.9132, 35.6024) (-17.9103, 35.5977) (-17.9075, 35.593) (-17.9047, 35.5884) (-17.9019, 35.5839) (-17.8991, 35.5794) (-17.8964, 35.575) (-17.8937, 35.5706) (-17.891, 35.5664) (-17.8883, 35.5621) (-17.8857, 35.558) (-17.8831, 35.5539) (-17.8806, 35.5499) (-17.8781, 35.5459) (-17.8756, 35.542) (-17.8731, 35.5382) (-17.8707, 35.5344) (-17.8683, 35.5308) (-17.866, 35.5271) (-17.8637, 35.5236) (-17.8614, 35.5201) (-17.8592, 35.5167) (-17.857, 35.5134) (-17.8548, 35.5101) (-17.8527, 35.5069) (-17.8506, 35.5038) (-17.8485, 35.5007) (-17.8465, 35.4978) (-17.8446, 35.4948) (-17.8427, 35.492) (-17.8408, 35.4893) (-17.8389, 35.4866) (-17.8372, 35.484) (-17.8354, 35.4814) (-17.8337, 35.479) (-17.8321, 35.4766) (-17.8305, 35.4743) (-17.8289, 35.4721) (-17.8274, 35.4699) (-17.826, 35.4679) (-17.8246, 35.4659) (-17.8232, 35.464) (-17.8219, 35.4622) (-17.8207, 35.4604) (-17.8195, 35.4588) (-17.8183, 35.4572) (-17.8172, 35.4557) (-17.8162, 35.4543) (-17.8153, 35.453) (-17.8144, 35.4518) (-17.8135, 35.4506) (-17.8127, 35.4496) (-17.812, 35.4486) (-17.8114, 35.4477) (-17.8108, 35.4469) (-17.8103, 35.4463) (-17.8098, 35.4457) (-17.8095, 35.4453) (-17.8093, 35.445) (-17.8092, 35.4448) (-17.8091, 35.4448) knots -1 -1 -1 -1 -1 -1 -0.99583333 -0.99166667 -0.9875 -0.98333333 -0.97916667 -0.975 -0.97083333 -0.96666667 -0.9625 -0.95833333 -0.95416667 -0.95 -0.94583333 -0.94166667 -0.9375 -0.93333333 -0.92916667 -0.925 -0.92083333 -0.91666667 -0.9125 -0.90833333 -0.90416667 -0.9 -0.89583333 -0.89166667 -0.8875 -0.88333333 -0.87916667 -0.875 -0.87083333 -0.86666667 -0.8625 -0.85833333 -0.85416667 -0.85 -0.84583333 -0.84166667 -0.8375 -0.83333333 -0.82916667 -0.825 -0.82083333 -0.81666667 -0.8125 -0.80833333 -0.80416667 -0.8 -0.79583333 -0.79166667 -0.7875 -0.78333333 -0.77916667 -0.775 -0.77083333 -0.76666667 -0.7625 -0.75833333 -0.75416667 -0.75 -0.74583333 -0.74166667 -0.7375 -0.73333333 -0.72916667 -0.725 -0.72083333 -0.71666667 -0.7125 -0.70833333 -0.70416667 -0.7 -0.69583333 -0.69166667 -0.6875 -0.68333333 -0.67916667 -0.675 -0.67083333 -0.66666667 -0.6625 -0.65833333 -0.65416667 -0.65 -0.64583333 -0.64166667 -0.6375 -0.63333333 -0.62916667 -0.625 -0.62083333 -0.61666667 -0.6125 -0.60833333 -0.60416667 -0.6 -0.59583333 -0.59166667 -0.5875 -0.58333333 -0.57916667 -0.575 -0.57083333 -0.56666667 -0.5625 -0.55833333 -0.55416667 -0.55 -0.54583333 -0.54166667 -0.5375 -0.53333333 -0.52916667 -0.525 -0.52083333 -0.51666667 -0.5125 -0.50833333 -0.50416667 -0.5 -0.49583333 -0.49166667 -0.4875 -0.48333333 -0.47916667 -0.475 -0.47083333 -0.46666667 -0.4625 -0.45833333 -0.45416667 -0.45 -0.44583333 -0.44166667 -0.4375 -0.43333333 -0.42916667 -0.425 -0.42083333 -0.41666667 -0.4125 -0.40833333 -0.40416667 -0.4 -0.39583333 -0.39166667 -0.3875 -0.38333333 -0.37916667 -0.375 -0.37083333 -0.36666667 -0.3625 -0.35833333 -0.35416667 -0.35 -0.34583333 -0.34166667 -0.3375 -0.33333333 -0.32916667 -0.325 -0.32083333 -0.31666667 -0.3125 -0.30833333 -0.30416667 -0.3 -0.29583333 -0.29166667 -0.2875 -0.28333333 -0.27916667 -0.275 -0.27083333 -0.26666667 -0.2625 -0.25833333 -0.25416667 -0.25 -0.24583333 -0.24166667 -0.2375 -0.23333333 -0.22916667 -0.225 -0.22083333 -0.21666667 -0.2125 -0.20833333 -0.20416667 -0.2 -0.19583333 -0.19166667 -0.1875 -0.18333333 -0.17916667 -0.175 -0.17083333 -0.16666667 -0.1625 -0.15833333 -0.15416667 -0.15 -0.14583333 -0.14166667 -0.1375 -0.13333333 -0.12916667 -0.125 -0.12083333 -0.11666667 -0.1125 -0.10833333 -0.10416667 -0.1 -0.09583333 -0.09166667 -0.0875 -0.08333333 -0.07916667 -0.075 -0.07083333 -0.06666667 -0.0625 -0.05833333 -0.05416667 -0.05 -0.04583333 -0.04166667 -0.0375 -0.03333333 -0.02916667 -0.025 -0.02083333 -0.01666667 -0.0125 -0.00833333 -0.00416667 0 0 0 0 0 0